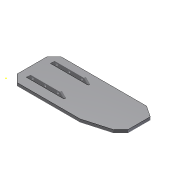
# Autodesk Inventor part: Right foot
Saved by Autodesk Inventor 2011 (Build 150239000, 239)
## iProperties
Created: 2010-11-21
Part Number: Right foot
Document SubType Name: Modeling
Designer: Milton
Density: 1 g/cm^3
Mass: 32.7853 g
Surface Area: 183.661 cm^2
Volume: 32.7853 cm^3
Author: Milton
Autodesk Inventor part; units mm, degrees
ref_plane "YZ Plane" through (0, 0, 0) normal (1, 0, 0) x (0, 1, 0)
ref_plane "XZ Plane" through (0, 0, 0) normal (0, 1, 0) x (-1, 0, 0)
ref_plane "XY Plane" through (0, 0, 0) normal (0, 0, 1) x (1, 0, 0)
sketch "Sketch1" plane through (0, 0, 0) normal (0, 0, 1) x (1, 0, 0)
  line L0 (2.4256, 52.3404) -> (2.4256, 12.3404)
  line L1 (12.4256, 2.3404) -> (97.4256, 2.3404)
  line L2 (142.4256, 22.3404) -> (142.4256, 52.3404)
  line L3 (127.4256, 62.3404) -> (12.4256, 62.3404)
  line L4 (2.4256, 52.3404) -> (12.4256, 62.3404)
  line L5 (97.4256, 2.3404) -> (132.4256, 12.3404)
  line L6 (2.4256, 12.3404) -> (12.4256, 2.3404)
  line L7 (142.4256, 22.3404) -> (132.4256, 12.3404)
  line L8 (127.4256, 62.3404) -> (142.4256, 52.3404)
  line L9 (12.4256, 49.8404) -> (12.4256, 47.3404)
  line L10 (63.4256, 49.8404) -> (63.4256, 47.3404)
  line L11 (12.4256, 47.3404) -> (63.4256, 47.3404)
  line L12 (63.4256, 47.3404) -> (63.4256, 49.8404)
  line L13 (63.4256, 49.8404) -> (12.4256, 49.8404)
  line L14 (12.4256, 14.8404) -> (12.4256, 17.3404)
  line L15 (63.4256, 14.8404) -> (63.4256, 17.3404)
  line L16 (12.4256, 17.3404) -> (63.4256, 17.3404)
  line L17 (63.4256, 17.3404) -> (63.4256, 14.8404)
  line L18 (63.4256, 14.8404) -> (12.4256, 14.8404)
  point P0 (0, 0)
  dimension "d14" = 140
  dimension "d15" = 10
  dimension "d16" = 10
  dimension "d17" = 51
  dimension "d18" = 51
  constraints: 38 end point
  measures "d14" distance between parallel lines of L2 L0
  measures "d15" distance between parallel lines of L0 L9
  measures "d16" distance between parallel lines of L0 L14
  measures "d17" distance between parallel lines of L10 L9
  measures "d18" distance between parallel lines of L15 L14
extrude "Extrusion1" add sketch "Sketch1" against normal blind 4 contours L4 L3 L8 L2 L7 L5 L1 L6 L0 | L13 L10 L11 L9 | L14 L16 L15 L18
extrude "Extrusion2" add sketch "Sketch1" along normal blind 5.6 contours L13 L10 L11 L9 | L14 L16 L15 L18
sketch "Sketch2" plane through (12.4256, 14.8404, 5.6) normal (0, -1, 0) x (1, 0, 0)
  line L0 (0, -5.6) -> (0, 0) projected
  line L1 (51, -5.6) -> (51, 0) projected
  circle A0 centre (8.5, -2.8) radius 1.35
  circle A1 centre (25.5, -2.8) radius 1.35
  circle A2 centre (42.5, -2.8) radius 1.35
  point P0 (50.8, -5.6)
  point P1 (-12.4256, -5.6)
  dimension "d5" = 2.7
  dimension "d6" = 8.5
  dimension "d7" = 2.7
  dimension "d8" = 2.7
  dimension "d9" = 8.5
  dimension "d10" = 17
  constraints: 3 centre point, 1 other
  measures "d5" diameter of A0
  measures "d6" distance from line of A0.centre L0
  measures "d7" diameter of A1
  measures "d8" diameter of A2
  measures "d10" distance of A2.centre A1.centre
extrude "Extrusion3" cut sketch "Sketch2" against normal through all
chamfer "Chamfer1" distance 5.6 angle 45 4 edges at (12.4256, 16.0904, 5.6) (63.4256, 48.5904, 5.6) (63.4256, 16.0904, 5.6) (12.4256, 48.5904, 5.6)
body "Solid1"
